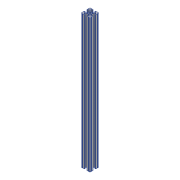
# Autodesk Inventor part: 20-006-20x20x550mm
Saved by Autodesk Inventor 2018.1 (Build 221171000, 171)
## iProperties
Created: 2017-08-13
Part Number: 20-006-20x20x550mm
Material: Aluminium 6061
Document SubType Name: Modeling
Designer: feesmrt
Density: 2.7 g/cm^3
Appearance: Aluminium - flach
Author: feesmrt
Autodesk Inventor part; units mm, degrees
ref_plane "YZ Plane" through (0, 0, 0) normal (1, 0, 0) x (0, 1, 0)
ref_plane "XZ Plane" through (0, 0, 0) normal (0, 1, 0) x (-1, 0, 0)
ref_plane "XY Plane" through (0, 0, 0) normal (0, 0, 1) x (1, 0, 0)
derived "Vorlage_Aluprofile_30x30.ipt"
sketch "Profil_Skizze" plane through (9.5, -15, 0) normal (0, 0, -1) x (-1, 0, 0)
  line L0 (14.3083, 18.677) -> (12.4023, 16.771)
  arc A0 (12.4023, 13.229) -> (12.4023, 16.771) centre (9.5, 15) ccw
  line L1 (12.4023, 13.229) -> (14.3083, 11.323)
  line L2 (14.3083, 11.323) -> (13.177, 10.1917)
  line L3 (13.177, 10.1917) -> (11.271, 12.0977)
  arc A1 (7.729, 12.0977) -> (11.271, 12.0977) centre (9.5, 15) ccw
  line L4 (7.729, 12.0977) -> (5.823, 10.1917)
  line L5 (5.823, 10.1917) -> (4.6917, 11.323)
  line L6 (4.6917, 11.323) -> (6.5977, 13.229)
  arc A2 (6.5977, 16.771) -> (6.5977, 13.229) centre (9.5, 15) ccw
  line L7 (6.5977, 16.771) -> (4.6917, 18.677)
  line L8 (4.6917, 18.677) -> (5.823, 19.8083)
  line L9 (5.823, 19.8083) -> (7.729, 17.9023)
  arc A3 (11.271, 17.9023) -> (7.729, 17.9023) centre (9.5, 15) ccw
  line L10 (11.271, 17.9023) -> (13.177, 19.8083)
  line L11 (13.177, 19.8083) -> (14.3083, 18.677)
  arc A4 (-3.5, 30) -> (-5.5, 28) centre (-3.5, 28) ccw
  line L12 (-5.5, 28) -> (-5.5, 25.5)
  line L13 (-5, 25) -> (-5.5, 25.5)
  line L14 (-5.5, 24.5) -> (-5, 25)
  line L15 (-5.5, 19.5) -> (-5.5, 24.5)
  line L16 (-5, 19.5) -> (-5.5, 19.5)
  line L17 (-5, 19) -> (-5, 19.5)
  line L18 (-2.7, 19) -> (-5, 19)
  line L19 (-2.7, 23) -> (-2.7, 19)
  arc A5 (-0.9929, 23.7071) -> (-2.7, 23) centre (-1.7, 23) ccw
  line L20 (-0.9929, 23.7071) -> (3.5, 19.2142)
  line L21 (3.5, 19.2142) -> (3.5, 15.3125)
  line L22 (3.8, 15) -> (3.5, 15.3125)
  line L23 (3.5, 14.6875) -> (3.8, 15)
  line L24 (3.5, 14.6875) -> (3.5, 10.7858)
  line L25 (-0.9929, 6.2929) -> (3.5, 10.7858)
  arc A6 (-2.7, 7) -> (-0.9929, 6.2929) centre (-1.7, 7) ccw
  line L26 (-2.7, 7) -> (-2.7, 11)
  line L27 (-5, 11) -> (-2.7, 11)
  line L28 (-5, 10.5) -> (-5, 11)
  line L29 (-5.5, 10.5) -> (-5, 10.5)
  line L30 (-5.5, 5.5) -> (-5.5, 10.5)
  line L31 (-5, 5) -> (-5.5, 5.5)
  line L32 (-5.5, 4.5) -> (-5, 5)
  line L33 (-5.5, 4.5) -> (-5.5, 2)
  arc A7 (-5.5, 2) -> (-3.5, 0) centre (-3.5, 2) ccw
  line L34 (-3.5, 0) -> (-1, 0)
  line L35 (-0.5, 0.5) -> (-1, 0)
  line L36 (0, 0) -> (-0.5, 0.5)
  line L37 (5, 0) -> (0, 0)
  line L38 (5, 0.5) -> (5, 0)
  line L39 (5.5, 0.5) -> (5, 0.5)
  line L40 (5.5, 2.8) -> (5.5, 0.5)
  line L41 (1.5, 2.8) -> (5.5, 2.8)
  arc A8 (0.7929, 4.5071) -> (1.5, 2.8) centre (1.5, 3.8) ccw
  line L42 (0.7929, 4.5071) -> (5.2858, 9)
  line L43 (5.2858, 9) -> (9.1875, 9)
  line L44 (9.5, 9.3) -> (9.1875, 9)
  line L45 (9.8125, 9) -> (9.5, 9.3)
  line L46 (9.8125, 9) -> (13.7142, 9)
  line L47 (18.2071, 4.5071) -> (13.7142, 9)
  arc A9 (17.5, 2.8) -> (18.2071, 4.5071) centre (17.5, 3.8) ccw
  line L48 (17.5, 2.8) -> (13.5, 2.8)
  line L49 (13.5, 0.5) -> (13.5, 2.8)
  line L50 (14, 0.5) -> (13.5, 0.5)
  line L51 (14, 0) -> (14, 0.5)
  line L52 (19, 0) -> (14, 0)
  line L53 (19.4899, 0.5) -> (19, 0)
  line L54 (19.9899, 0) -> (19.4899, 0.5)
  line L55 (19.9899, 0) -> (22.5, 0)
  arc A10 (22.5, 0) -> (24.5, 2) centre (22.5, 2) ccw
  line L56 (24.5, 2) -> (24.5, 4.5)
  line L57 (24, 5) -> (24.5, 4.5)
  line L58 (24.5, 5.5) -> (24, 5)
  line L59 (24.5, 5.5) -> (24.5, 10.5)
  line L60 (24, 10.5) -> (24.5, 10.5)
  line L61 (24, 11) -> (24, 10.5)
  line L62 (21.7, 11) -> (24, 11)
  line L63 (21.7, 7) -> (21.7, 11)
  arc A11 (19.9929, 6.2929) -> (21.7, 7) centre (20.7, 7) ccw
  line L64 (19.9929, 6.2929) -> (15.5, 10.7858)
  line L65 (15.5, 10.7858) -> (15.5, 14.6875)
  line L66 (15.2, 15) -> (15.5, 14.6875)
  line L67 (15.5, 15.3125) -> (15.2, 15)
  line L68 (15.5, 15.3125) -> (15.5, 19.2142)
  line L69 (19.9929, 23.7071) -> (15.5, 19.2142)
  arc A12 (21.7, 23) -> (19.9929, 23.7071) centre (20.7, 23) ccw
  line L70 (21.7, 19) -> (21.7, 23)
  line L71 (24, 19) -> (21.7, 19)
  line L72 (24, 19.5) -> (24, 19)
  line L73 (24.5, 19.5) -> (24, 19.5)
  line L74 (24.5, 19.5) -> (24.5, 24.5)
  line L75 (24, 25) -> (24.5, 24.5)
  line L76 (24.5, 25.5) -> (24, 25)
  line L77 (24.5, 25.5) -> (24.5, 28)
  arc A13 (24.5, 28) -> (22.5, 30) centre (22.5, 28) ccw
  line L78 (22.5, 30) -> (20, 30)
  line L79 (19.5, 29.5) -> (20, 30)
  line L80 (19, 30) -> (19.5, 29.5)
  line L81 (19, 30) -> (14, 30)
  line L82 (14, 29.5) -> (14, 30)
  line L83 (13.5, 29.5) -> (14, 29.5)
  line L84 (13.5, 27.2) -> (13.5, 29.5)
  line L85 (17.5, 27.2) -> (13.5, 27.2)
  arc A14 (18.2071, 25.4929) -> (17.5, 27.2) centre (17.5, 26.2) ccw
  line L86 (18.2071, 25.4929) -> (13.7142, 21)
  line L87 (13.7142, 21) -> (9.8125, 21)
  line L88 (9.5, 20.7) -> (9.8125, 21)
  line L89 (9.1875, 21) -> (9.5, 20.7)
  line L90 (9.1875, 21) -> (5.2858, 21)
  line L91 (0.7929, 25.4929) -> (5.2858, 21)
  arc A15 (1.5, 27.2) -> (0.7929, 25.4929) centre (1.5, 26.2) ccw
  line L92 (5.5, 27.2) -> (1.5, 27.2)
  line L93 (5.5, 29.5) -> (5.5, 27.2)
  line L94 (5, 29.5) -> (5.5, 29.5)
  line L95 (5, 30) -> (5, 29.5)
  line L96 (5, 30) -> (0, 30)
  line L97 (-0.5, 29.5) -> (0, 30)
  line L98 (-1, 30) -> (-0.5, 29.5)
  line L99 (-1, 30) -> (-3.5, 30)
extrude "Extrusion1" add sketch "Profil_Skizze" along normal mid plane 450
